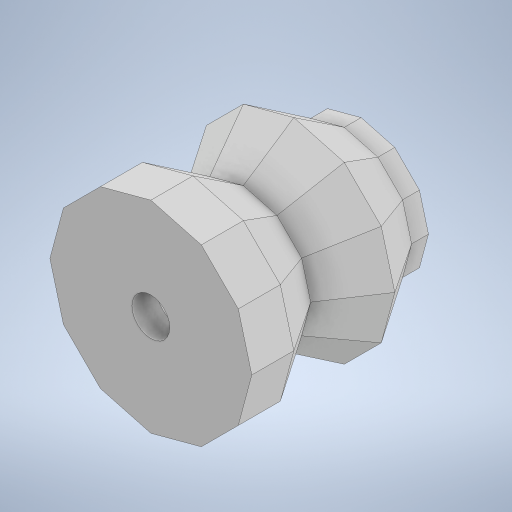
# Autodesk Inventor part: Test12
Saved by Autodesk Inventor 2023 (Build 270158000, 158)
## iProperties
Created: 2024-07-03
Part Number: Test12
Material: 일반
Document SubType Name: Modeling
Designer: ojs08
Density: 1 g/cm^3
Appearance: 기본값
Author: ojs08
Autodesk Inventor part; units mm, degrees
ref_plane "YZ Plane" through (0, 0, 0) normal (1, 0, 0) x (0, 1, 0)
ref_plane "XZ Plane" through (0, 0, 0) normal (0, 1, 0) x (-1, 0, 0)
sketch "스케치1" plane through (0, 0, 0) normal (0, 0, 1) x (1, 0, 0)
  line L0 (10.3923, 6) -> (12, 0)
  line L1 (12, 0) -> (10.3923, -6)
  line L2 (10.3923, -6) -> (6, -10.3923)
  line L3 (6, -10.3923) -> (0, -12)
  line L4 (0, -12) -> (-6, -10.3923)
  line L5 (-6, -10.3923) -> (-10.3923, -6)
  line L6 (-10.3923, -6) -> (-12, 0)
  line L7 (-12, 0) -> (-10.3923, 6)
  line L8 (-10.3923, 6) -> (-6, 10.3923)
  line L9 (-6, 10.3923) -> (0, 12)
  line L10 (0, 12) -> (6, 10.3923)
  line L11 (6, 10.3923) -> (10.3923, 6)
  line L12 (-16.8, 0) -> (16.8, 0) projected
  point P0 (0, 0)
  point P1 (0, 0)
  dimension "d0" = 24
  constraints: 24 end point, 1 coincident, 1 point on line, 25 other
  measures "d0" distance of L0.end L6.end
ref_plane "작업 평면1" through (0, 0, 6) normal (0, 0, 1) x (1, 0, 0)
sketch "스케치2" plane through (0, 0, 6) normal (0, 0, 1) x (1, 0, 0)
  line L0 (6.9282, 4) -> (8, 0)
  line L1 (8, 0) -> (6.9282, -4)
  line L2 (6.9282, -4) -> (4, -6.9282)
  line L3 (4, -6.9282) -> (0, -8)
  line L4 (0, -8) -> (-4, -6.9282)
  line L5 (-4, -6.9282) -> (-6.9282, -4)
  line L6 (-6.9282, -4) -> (-8, 0)
  line L7 (-8, 0) -> (-6.9282, 4)
  line L8 (-6.9282, 4) -> (-4, 6.9282)
  line L9 (-4, 6.9282) -> (0, 8)
  line L10 (0, 8) -> (4, 6.9282)
  line L11 (4, 6.9282) -> (6.9282, 4)
  line L12 (-16.8, 0) -> (16.8, 0) projected
  point P0 (0, 0)
  point P1 (0, 0)
  dimension "d2" = 16
  constraints: 24 end point, 1 coincident, 1 point on line, 25 other
  measures "d2" distance of L0.end L6.end
loft "로프트1" add profiles "스케치1", "스케치2"
mirror "미러1" about plane through (0, 0, 6) normal (0, 0, 1) of "로프트1"
mirror "미러2" about plane through (0, 0, 0) normal (0, 0, -1) of "로프트1"
sketch "스케치3" plane through (12, 0, 12) normal (0, 0, 1) x (0.9659258, 0.258819, 0)
  line L0 (0, 6.2117) -> (0, 0) projected
  line L1 (-3.1058, 11.5911) -> (0, 6.2117) projected
  line L2 (-8.4853, 14.6969) -> (-3.1058, 11.5911) projected
  line L3 (-14.6969, 14.6969) -> (-8.4853, 14.6969) projected
  line L4 (-20.0764, 11.5911) -> (-14.6969, 14.6969) projected
  line L5 (-23.1822, 6.2117) -> (-20.0764, 11.5911) projected
  line L6 (-23.1822, 0) -> (-23.1822, 6.2117) projected
  line L7 (-20.0764, -5.3795) -> (-23.1822, 0) projected
  line L8 (-14.6969, -8.4853) -> (-20.0764, -5.3795) projected
  line L9 (-8.4853, -8.4853) -> (-14.6969, -8.4853) projected
  line L10 (-3.1058, -5.3795) -> (-8.4853, -8.4853) projected
  line L11 (0, 0) -> (-3.1058, -5.3795) projected
  point P0 (-11.5911, 3.1058)
extrude "돌출1" add sketch "스케치3" along normal blind 2.5
shell "쉘1" thickness 0.5 removed faces 0 ; own thickness 2 on faces at (-7.9362, 6.6348, -2) (-3.5556, 9.714, -2) (1.7778, 10.1903, -2) (6.6348, 7.9362, -2) (9.714, 3.5556, -2) (10.1903, -1.7778, -2) (7.9362, -6.6348, -2) (3.5556, -9.714, -2) (-1.7778, -10.1903, -2) (-6.6348, -7.9362, -2) (-9.714, -3.5556, -2) (-10.1903, 1.7778, -2) (6.6348, 7.9362, 10) (1.7778, 10.1903, 10) (-3.5556, 9.714, 10) (-7.9362, 6.6348, 10) (9.714, 3.5556, 10) (10.1903, -1.7778, 10) (7.9362, -6.6348, 10) (3.5556, -9.714, 10) (-10.1903, 1.7778, 10) (-9.714, -3.5556, 10) (-6.6348, -7.9362, 10) (-1.7778, -10.1903, 10)
sketch "스케치4" plane through (12, 0, 14.5) normal (0, 0, 1) x (0.9659258, 0.258819, 0)
  line L0 (-3.1058, 11.5911) -> (-8.4853, 14.6969) projected
  line L1 (-8.4853, 14.6969) -> (-14.6969, 14.6969) projected
  line L2 (-14.6969, 14.6969) -> (-20.0764, 11.5911) projected
  line L3 (-20.0764, 11.5911) -> (-23.1822, 6.2117) projected
  line L4 (-23.1822, 6.2117) -> (-23.1822, 0) projected
  line L5 (-23.1822, 0) -> (-20.0764, -5.3795) projected
  line L6 (-20.0764, -5.3795) -> (-14.6969, -8.4853) projected
  line L7 (-14.6969, -8.4853) -> (-8.4853, -8.4853) projected
  line L8 (-8.4853, -8.4853) -> (-3.1058, -5.3795) projected
  line L9 (-3.1058, -5.3795) -> (0, 0) projected
  line L10 (0, 0) -> (0, 6.2117) projected
  line L11 (0, 6.2117) -> (-3.1058, 11.5911) projected
  point P0 (-11.5911, 3.1058)
extrude "돌출2" add sketch "스케치4" along normal blind 2.5
sketch "스케치5" plane through (12, 0, 17) normal (0, 0, 1) x (0.9659258, 0.258819, 0)
  circle A0 centre (-11.5911, 3.1058) radius 2.25
  point P0 (-11.5911, 3.1058)
  dimension "d13" = 4.5
  constraints: 1 centre point, 1 coincident
  measures "d13" diameter of A0
extrude "돌출3" cut sketch "스케치5" against normal blind 3
sketch "스케치6" plane through (8, 0, -6) normal (0, 0, -1) x (-0.9659258, -0.258819, 0)
  line L0 (0, 4.1411) -> (0, 0) projected
  line L1 (0, 0) -> (2.0706, -3.5863) projected
  line L2 (2.0706, -3.5863) -> (5.6569, -5.6569) projected
  line L3 (5.6569, -5.6569) -> (9.798, -5.6569) projected
  line L4 (9.798, -5.6569) -> (13.3843, -3.5863) projected
  line L5 (13.3843, -3.5863) -> (15.4548, 0) projected
  line L6 (15.4548, 0) -> (15.4548, 4.1411) projected
  line L7 (15.4548, 4.1411) -> (13.3843, 7.7274) projected
  line L8 (13.3843, 7.7274) -> (9.798, 9.798) projected
  line L9 (9.798, 9.798) -> (5.6569, 9.798) projected
  line L10 (5.6569, 9.798) -> (2.0706, 7.7274) projected
  line L11 (2.0706, 7.7274) -> (0, 4.1411) projected
  point P0 (7.7274, 2.0706)
extrude "돌출4" add sketch "스케치6" along normal blind 2
